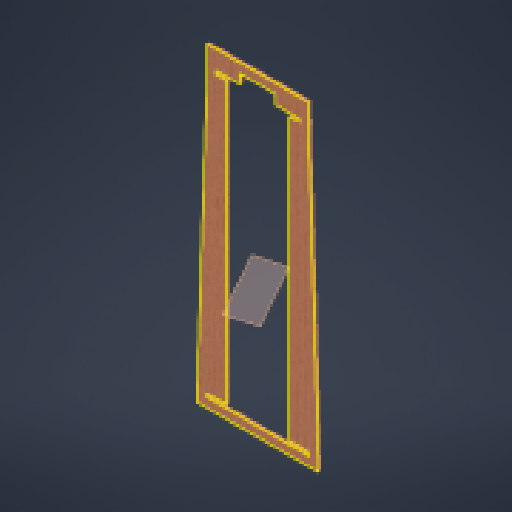
# Autodesk Inventor part: Upper Stand Bracket
Saved by Autodesk Inventor 2025.2 (Build 292293000, 293)
## iProperties
Created: 2024-11-19
Part Number: Upper Stand Bracket
Material: Wood (Oak)
Document SubType Name: Modeling
Designer: JL
Density: 0.76 g/cm^3
Appearance: White Oak - Natural Medium Gloss
Author: JL
Autodesk Inventor part; units mm, degrees
ref_plane "YZ Plane" through (0, 0, 0) normal (1, 0, 0) x (0, 1, 0)
ref_plane "XZ Plane" through (0, 0, 0) normal (0, 1, 0) x (-1, 0, 0)
ref_plane "XY Plane" through (0, 0, 0) normal (0, 0, 1) x (1, 0, 0)
ref_plane "Work Plane1" through (-10, 297.2462, 0) normal (0, 0, 1) x (0, -1, 0)
ref_plane "Work Plane2" through (-53.2, 294.1262, 848.1435) normal (1, 0, 0) x (0, 0.6133, 0.7899)
sketch "Sketch1" plane through (-10, 297.2462, 0) normal (0, 0, 1) x (0, -1, 0)
  line L0 (94.5216, -24.7) -> (0, -24.7) projected
  line L1 (0, 0) -> (0, -24.7) projected
  line L2 (0, 0) -> (307.2462, 0) projected
  line L3 (307.2462, -10.6) -> (307.2462, 0) projected
  line L4 (307.2462, -10.6) -> (94.5216, -10.6) projected
  line L5 (94.5216, -10.6) -> (94.5216, -24.7) projected
  line L6 (89.5216, -75.8) -> (297.2462, -75.8) projected
  line L7 (297.2462, -75.8) -> (297.2462, -10.6) projected
  line L8 (307.2462, -10.6) -> (297.2462, -10.6) projected
  line L9 (307.2462, -10.6) -> (307.2462, -86.4) projected
  line L10 (0, -86.4) -> (307.2462, -86.4) projected
  line L11 (0, -86.4) -> (0, -61.7) projected
  line L12 (89.5216, -61.7) -> (0, -61.7) projected
  line L13 (89.5216, -75.8) -> (89.5216, -61.7) projected
  line L14 (297.2462, 10) -> (294.2462, 10) projected
  line L15 (297.2462, 10) -> (297.2462, 20) projected
  line L16 (297.2462, 20) -> (294.2462, 20) projected
  line L17 (294.2462, 10) -> (294.2462, 20) projected
  line L18 (297.2462, 10) -> (294.2462, 10) projected
  line L19 (0, 0) -> (0, 10) projected
  line L20 (0, 10) -> (-3, 10) projected
  line L21 (-3, 0) -> (-3, 10) projected
  line L22 (0, 0) -> (-3, 0) projected
  line L23 (0, -24.7) -> (-3, -24.7) projected
  line L24 (307.2462, 0) -> (307.2462, 20)
  line L25 (307.2462, 20) -> (297.2462, 20)
  line L26 (294.2462, 20) -> (0, 10)
  line L27 (-13, -24.7) -> (-3, -24.7)
  line L28 (-3, -24.7) -> (-3, 0)
  line L29 (-3, 10) -> (-13, 10)
  line L30 (-13, 10) -> (-13, -24.7)
  line L31 (297.2462, -43.2) -> (307.2462, -43.2)
  line L32 (297.2462, 10) -> (297.2462, -10.6)
  line L33 (294.2462, 10) -> (294.2462, -10.6)
  line L34 (94.5216, -10.6) -> (0, -10.6)
  line L35 (-89.0492, -43.2) -> (373.2954, -43.2) construction
  line L36 (-13, 10) -> (-23, 10)
  line L37 (-23, 10) -> (-23, -43.2)
  line L38 (-13, -24.7) -> (-13, -43.2)
  line L39 (-23, -43.2) -> (-13, -43.2)
  line L40 (297.4962, 10.25) -> (297.4962, -43.2)
  line L41 (297.4962, 10.25) -> (293.9962, 10.25)
  line L42 (293.9962, 10.25) -> (293.9962, -10.6)
  line L43 (0.25, 0.25) -> (0.25, -24.7)
  line L44 (-3.25, 0.25) -> (-3.25, -24.7)
  line L45 (-3.25, 0.25) -> (0.25, 0.25)
  point P0 (-3, 0.25)
  point P1 (0, 0.25)
  point P2 (0.25, -10.6)
  point P3 (297.4962, -43.2)
  dimension "d1" = 10
  dimension "d2" = 10
  dimension "d5" = 0.25
  dimension "d6" = 0.25
  dimension "d7" = 0.25
  dimension "d8" = 0.25
  dimension "d9" = 0.25
  dimension "d10" = 0.25
  constraints: 42 end point, 9 point on line, 8 perpendicular, 5 parallel, 2 collinear, 2 horizontal, 1 midpoint, 1 vertical
  measures "d1" distance of L20.end L29.end
  measures "d2" distance of L29.end L36.end
  measures "d5" distance between parallel lines of L32 L40
  measures "d6" distance between parallel lines of L14 L41
  measures "d7" distance between parallel lines of L33 L42
  measures "d8" distance between parallel lines of L1 L43
  measures "d9" distance between parallel lines of L28 L44
  measures "d10" distance between parallel lines of L22 L45
extrude "Extrusion1" add sketch "Sketch1" along normal blind 3 contours L34 L43 L2 L42 L4 | L43 L45 L19 L26 L17 L41 L42 L2 | L27 L30 L29 L21 L45 L44 | L45 L21 L20 L19 | L38 L39 L37 L36 L30 | L40 L2 L3 L4 | L4 L9 L31 L40 | L17 L16 L15 L41 | L40 L41 L15 L25 L24 L2
mirror "Mirror1" about plane through (-53.2, 294.1262, 848.1435) normal (1, 0, 0)
sketch "Sketch2" plane through (-10, 297.2462, 3) normal (0, 0, 1) x (1, 0, 0)
  line L0 (20, -307.2462) -> (-106.4, -307.2462) projected
  line L1 (20, -307.2462) -> (20, -294.2462) projected
  line L2 (20, -294.2462) -> (10, 0) projected
  line L3 (10, 0) -> (10, 23) projected
  line L4 (10, 23) -> (-96.4, 23) projected
  line L5 (-96.4, 0) -> (-96.4, 23) projected
  line L6 (-106.4, -294.2462) -> (-96.4, 0) projected
  line L7 (-106.4, -307.2462) -> (-106.4, -294.2462) projected
  line L8 (-75.8, -0.25) -> (-75.8, -293.9962) projected
  line L9 (-61.7, 13) -> (-61.7, 3.25) projected
  line L10 (-24.7, 13) -> (-61.7, 13) projected
  line L11 (-24.7, 13) -> (-24.7, 3.25) projected
  line L12 (-10.6, -0.25) -> (-10.6, -293.9962) projected
  line L13 (10.25, -297.4962) -> (-96.65, -297.4962) projected
  line L14 (-96.65, -293.9962) -> (-96.65, -297.4962) projected
  line L15 (-75.8, -293.9962) -> (-96.65, -293.9962) projected
  line L16 (-86.65, -0.25) -> (-75.8, -0.25) projected
  line L17 (-86.65, 3.25) -> (-86.65, -0.25) projected
  line L18 (-61.7, 3.25) -> (-86.65, 3.25) projected
  line L19 (-24.7, 3.25) -> (0.25, 3.25) projected
  line L20 (0.25, 3.25) -> (0.25, -0.25) projected
  line L21 (0.25, -0.25) -> (-10.6, -0.25) projected
  line L22 (-10.6, -293.9962) -> (10.25, -293.9962) projected
  line L23 (10.25, -293.9962) -> (10.25, -297.4962) projected
  point P0 (10, -297.2462)
equation "\"d6\" = d5"
equation "\"d7\" = d5"
equation "\"d8\" = d5"
equation "\"d9\" = d5"
equation "\"d10\" = d5"
body "Solid1"
